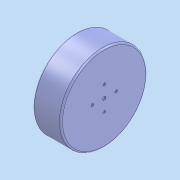
# Autodesk Inventor part: 바퀴
Saved by Autodesk Inventor 2020 (Build 240168000, 168)
## iProperties
Created: 2020-05-04
Part Number: 바퀴
Material: 일반
Document SubType Name: Modeling
Designer: sbahn
Density: 1 g/cm^3
Appearance: PTFE
Author: sbahn
Autodesk Inventor part; units mm, degrees
ref_plane "YZ Plane" through (0, 0, 0) normal (1, 0, 0) x (0, 1, 0)
ref_plane "XZ Plane" through (0, 0, 0) normal (0, 1, 0) x (-1, 0, 0)
ref_plane "XY Plane" through (0, 0, 0) normal (0, 0, 1) x (1, 0, 0)
sketch "스케치1" plane through (0, 0, 0) normal (1, 0, 0) x (0, 1, 0)
  circle A0 centre (0, 0) radius 55
  circle A1 centre (0, 0) radius 54
  dimension "d0" = 110
  dimension "d1" = 1
  constraints: 2 centre point, 1 coincident
  measures "d0" diameter of A0
  measures "d1" radial gap between concentric circles of A0 A1
extrude "돌출1" add sketch "스케치1" along normal mid plane 36
sketch "스케치2" plane through (18, 0, 0) normal (1, 0, 0) x (0, 0, -1)
  circle A0 centre (0, 0) radius 55 projected
  circle A1 centre (0, 0) radius 2
  dimension "d4" = 4
  constraints: 1 centre point, 1 coincident
  measures "d4" diameter of A1
extrude "돌출2" add sketch "스케치2" against normal blind 1
sketch "스케치3" plane through (-18, 0, 0) normal (-1, 0, 0) x (0, 0, 1)
  circle A0 centre (0, 0) radius 2 projected
  circle A1 centre (0, 0) radius 54 projected
extrude "돌출3" add sketch "스케치3" against normal blind 1
sketch "스케치4" plane through (-18, 0, 0) normal (-1, 0, 0) x (0, 0, 1)
  circle A0 centre (0, 0) radius 15.25
  line L0 (0, 0) -> (15.25, 0)
  circle A1 centre (15.25, 0) radius 1.5
  dimension "d9" = 30.5
  dimension "d10" = 3
  constraints: 2 coincident, 2 end point, 1 centre point, 1 horizontal, 1 horizontal alignment, 2 other
  measures "d10" diameter of A1
extrude "돌출4" cut sketch "스케치4" against normal blind 36 contours L0 A1 A0 | A0 A1 | A0 A1 L0 picked at (15.6947, -0.39)
pattern_circular "원형 패턴1" count 4 over 360 about axis through (-18, 0, 0) along (1, 0, 0) of "돌출4"
fillet "모깎기1" radius 2 3 edges at (18, 38.8909, -38.8909) (18, -38.8909, 38.8909) (-18, -55, 0)
